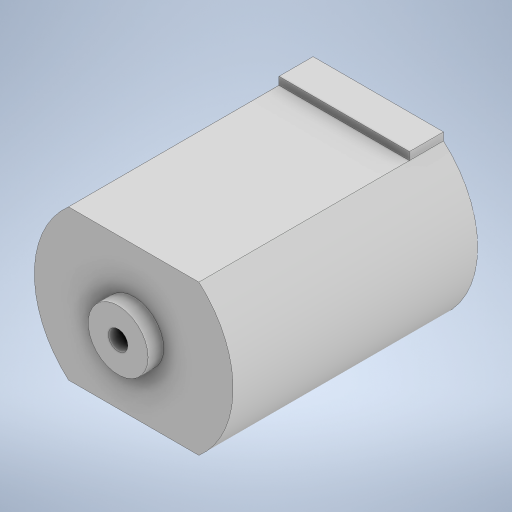
# Autodesk Inventor part: DCMotor
Saved by Autodesk Inventor 2023 (Build 270158000, 158)
## iProperties
Created: 2023-03-09
Part Number: DCMotor
Material: Generic
Document SubType Name: Modeling
Designer: czapa
Density: 1 g/cm^3
Appearance: Default
Author: czapa
Autodesk Inventor part; units mm, degrees
ref_plane "XZ Plane" through (0, 0, 0) normal (0, 1, 0) x (-1, 0, 0)
ref_plane "XY Plane" through (0, 0, 0) normal (0, 0, 1) x (1, 0, 0)
sketch "Sketch1" plane through (0, 0, 0) normal (0, 0, 1) x (1, 0, 0)
  circle A0 centre (0, 0) radius 10.2
  dimension "d0" = 20.4
  constraints: 1 centre point
  measures "d0" diameter of A0
extrude "Extrusion1" add sketch "Sketch1" along normal blind 25.1
ref_plane "Work Plane1" through (0, 0, 0) normal (1, 0, 0) x (0, 1, 0)
sketch "Sketch2" plane through (0, 0, 0) normal (1, 0, 0) x (0, 1, 0)
  line L0 (10.2, 25.1) -> (-10.2, 25.1) projected
  line L1 (10.2, 25.1) -> (-10.2, 25.1)
  line L2 (-10.2, 25.1) -> (-10.2, 0)
  line L3 (-10.2, 0) -> (10.2, 0)
  line L4 (10.2, 0) -> (10.2, 25.1)
  line L5 (0, 0) -> (7.7, 0)
  line L6 (7.7, 0) -> (7.7, 25.1)
  line L7 (7.7, 25.1) -> (0, 25.1)
  line L8 (0, 25.1) -> (0, 0)
  line L9 (10.2, 0) -> (-10.2, 0) projected
  line L10 (7.7, 25.1) -> (10.2, 25.1)
  line L11 (10.2, 25.1) -> (10.2, 0)
  line L12 (10.2, 0) -> (7.7, 0)
  line L13 (7.7, 0) -> (7.7, 25.1)
  line L14 (0, 25.1) -> (-7.7, 25.1)
  line L15 (-7.7, 25.1) -> (-7.7, 0)
  line L16 (-7.7, 0) -> (0, 0)
  line L17 (0, 0) -> (0, 25.1)
  line L18 (-7.7, 0) -> (-10.2, 0)
  line L19 (-10.2, 0) -> (-10.2, 25.1)
  line L20 (-10.2, 25.1) -> (-7.7, 25.1)
  line L21 (-7.7, 25.1) -> (-7.7, 0)
  dimension "d4" = 7.7
  dimension "d5" = 7.7
  constraints: 40 end point, 10 parallel, 5 horizontal, 5 perpendicular, 2 point on line
  measures "d4" distance of L7.end L6.end
  measures "d5" distance of L16.end L15.end
extrude "Extrusion2" cut sketch "Sketch2" along normal mid plane 22 contours L4 L3 L6 L0 | L15 L3 L2 L0
sketch "Sketch3" plane through (0, 0, 25.1) normal (0, 0, 1) x (1, 0, 0)
  circle A0 centre (0, 0) radius 3.075
  circle A1 centre (0, 0) radius 1
  dimension "d8" = 6.15
  dimension "d9" = 2
  constraints: 2 centre point, 2 coincident
  measures "d8" diameter of A0
  measures "d9" diameter of A1
extrude "Extrusion3" add sketch "Sketch3" along normal blind 1.6
sketch "Sketch4" plane through (-6.6895, 7.7, 25.1) normal (0, 1, 0) x (1, 0, 0)
  line L0 (0, 0) -> (0, 25.1) projected
  line L1 (13.3791, 25.1) -> (13.3791, 0) projected
  line L2 (0, 25.1) -> (13.3791, 25.1)
  line L3 (13.3791, 25.1) -> (13.3791, 21.6)
  line L4 (13.3791, 21.6) -> (0, 21.6)
  line L5 (0, 21.6) -> (0, 25.1)
  point P0 (6.6895, 25.1)
  dimension "d12" = 3.5
  constraints: 8 end point, 2 parallel, 1 horizontal, 1 perpendicular, 1 point on line
  measures "d12" distance of L2.end L3.end
extrude "Extrusion4" add sketch "Sketch4" along normal blind 0.8
sketch "Sketch5" plane through (0, 0, 0) normal (0, 0, -1) x (-1, 0, 0)
  circle A0 centre (0, 0) radius 4.75
  line L0 (-3.5382, -3.1691) -> (3.5382, -3.1691)
  dimension "d15" = 9.5
  constraints: 2 end point, 2 point on circle, 1 centre point, 1 coincident, 1 horizontal
  measures "d15" diameter of A0
extrude "Extrusion6" add sketch "Sketch5" along normal blind 1.6 contours A0 L0 picked at (0.1876, -0.5406)
body "Solid1"
